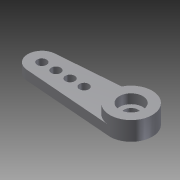
# Autodesk Inventor part: horn aluminium
Saved by Autodesk Inventor 2012 (Build 160160000, 160)
## iProperties
Created: 2013-12-06
Part Number: horn aluminium
Material: Default
Document SubType Name: Modeling
Designer: Irwan Haryanto
Density: 1 g/cm^3
Author: Irwan Haryanto
Autodesk Inventor part; units mm, degrees
ref_plane "YZ Plane" through (0, 0, 0) normal (1, 0, 0) x (0, 1, 0)
ref_plane "XZ Plane" through (0, 0, 0) normal (0, 1, 0) x (-1, 0, 0)
ref_plane "XY Plane" through (0, 0, 0) normal (0, 0, 1) x (1, 0, 0)
sketch "Sketch1" plane through (0, 0, 0) normal (0, 0, 1) x (1, 0, 0)
  circle A0 centre (-16, 0) radius 1
  circle A1 centre (-13, 0) radius 1
  circle A2 centre (0, 0) radius 1.5
  arc A3 (-19.2347, 2.9908) -> (-19.2347, -2.9908) centre (-19, 0) ccw
  arc A4 (-0.7018, -4.4449) -> (-0.7018, 4.4449) centre (0, 0) ccw
  line L0 (0, -4.5) -> (-19.2347, -2.9908)
  line L1 (0, 4.5) -> (-19.2347, 2.9908)
  dimension "d1" = 2
  dimension "d2" = 2
  dimension "d3" = 3
  dimension "d6" = 3
  dimension "d8" = 6
  dimension "d9" = 9
  dimension "d10" = 3
  constraints: 6 point on circle, 5 centre point, 4 end point, 2 point on line, 2 tangent, 1 coincident
  measures "d1" diameter of A0
  measures "d2" diameter of A1
  measures "d3" distance of A1.centre A0.centre
  measures "d6" diameter of A2
  measures "d8" diameter of A3
  measures "d9" diameter of A4
  measures "d10" distance of A0.centre A3.centre
extrude "Extrusion1" add sketch "Sketch1" along normal blind 2 contours L1 A4 L0 A3
sketch "Sketch2" plane through (0, 0, 2) normal (0, 0, 1) x (1, 0, 0)
  circle A0 centre (0, 0) radius 1.5 projected
  arc A1 (0, -4.5) -> (0, 4.5) centre (0, 0) ccw projected
  circle A2 centre (0, 0) radius 4.5
  dimension "d13" = 9
  constraints: 1 centre point, 1 coincident
  measures "d13" diameter of A2
extrude "Extrusion2" add sketch "Sketch2" along normal blind 2
sketch "Sketch3" plane through (0, 0, 4) normal (0, 0, 1) x (1, 0, 0)
  circle A0 centre (0, 0) radius 1.5 projected
  circle A1 centre (0, 0) radius 4.5 projected
  circle A2 centre (0, 0) radius 2.5
  dimension "d16" = 5
  constraints: 1 centre point, 1 coincident
  measures "d16" diameter of A2
hole "Hole1" at (0, 0, 4) direction (0, 0, -1) diameter 5 depth 2
sketch "Sketch4" plane through (0, 0, 2) normal (0, 0, 1) x (1, 0, 0)
  arc A0 (-19.2347, 2.9908) -> (-19.2347, -2.9908) centre (-19, 0) ccw projected
  circle A1 centre (-16, 0) radius 1 projected
  circle A2 centre (-13, 0) radius 1 projected
  circle A3 centre (-19, 0) radius 1
  circle A4 centre (-10, 0) radius 1
  dimension "d24" = 2
  dimension "d25" = 2
  dimension "d26" = 3
  dimension "d27" = 3
  constraints: 2 centre point, 1 coincident
  measures "d24" diameter of A3
  measures "d25" diameter of A4
  measures "d26" distance of A1.centre A3.centre
  measures "d27" distance of A2.centre A4.centre
hole "Hole2" at (-19, 0, 2) at (-10, 0, 2) direction (0, 0, -1) diameter 2 end through all
body "Solid1"
